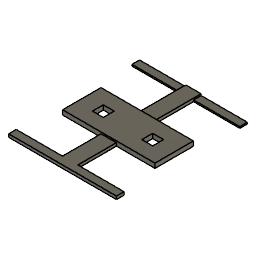
Ventilator Halterung andere Maße (Autodesk Fusion 360 design; units mm, degrees)
part number: 2026-08-07-16-50-58-000
Autodesk Fusion 360 part; units mm, degrees
sketch "Sketch1" plane through (0, 0, 0) normal (0, 0, 1) x (1, 0, 0)
  line L0 (0, 0) -> (60, 0)
  line L1 (60, 0) -> (60, 25)
  line L2 (60, 25) -> (0, 25)
  line L3 (0, 25) -> (0, 0)
  line L4 (5, 20) -> (55, 20)
  line L5 (55, 20) -> (55, 5)
  line L6 (55, 5) -> (5, 5)
  line L7 (5, 5) -> (5, 20)
  line L8 (10.5, 16) -> (17.5, 16)
  line L9 (17.5, 16) -> (17.5, 9)
  line L10 (17.5, 9) -> (10.5, 9)
  line L11 (10.5, 9) -> (10.5, 16)
  line L12 (42.5, 16) -> (49.5, 16)
  line L13 (49.5, 16) -> (49.5, 9)
  line L14 (49.5, 9) -> (42.5, 9)
  line L15 (42.5, 9) -> (42.5, 16)
  dimension "d1" = 60
  dimension "d2" = 25
  dimension "d3" = 50
  dimension "d4" = 15
  dimension "d5" = 5
  dimension "d7" = 5
  dimension "d8" = 7
  dimension "d9" = 7
  dimension "d10" = 4
  dimension "d12" = 7
  dimension "d13" = 7
  dimension "d15" = 4
  dimension "d16" = 5.5
  dimension "d17" = 5.5
  dimension "d18" = 25
  constraint horizontal L0
  constraint vertical L1
  constraint horizontal L2
  constraint vertical L3
  constraint coincident L0.start L3.end
  constraint horizontal L4
  constraint vertical L5
  constraint horizontal L6
  constraint vertical L7
  constraint horizontal L8
  constraint vertical L9
  constraint horizontal L10
  constraint vertical L11
  constraint horizontal L12
  constraint vertical L13
  constraint horizontal L14
  constraint vertical L15
  measures "d1" distance of L0.start L0.end
  measures "d2" distance of L0.start L2.end
  measures "d3" distance of L4.start L4.end
  measures "d4" distance of L4.start L6.end
  measures "d5" distance of L2 L4
  measures "d7" distance of L3 L7
  measures "d8" distance of L8.start L8.end
  measures "d9" distance of L8.start L10.end
  measures "d10" distance of L4 L8
  measures "d12" distance of L12.start L12.end
  measures "d13" distance of L12.start L14.end
  measures "d15" distance of L6 L14
  measures "d16" distance of L5 L13
  measures "d17" distance of L7 L11
  measures "d18" distance of L9 L15
sketch "Sketch2" plane through (0, 0, 0) normal (0, 0, 1) x (1, 0, 0)
extrude "Extrude1" add sketch "Sketch1" along normal blind 3 contours L0 L1 L2 L3 | L4 L5 L6 L7
sketch "Sketch3" plane through (0, 0, 0) normal (0, -1, 0) x (1, 0, 0)
  line L0 (0, 0) -> (60, 0)
  line L1 (60, 0) -> (60, 3)
  line L2 (60, 3) -> (0, 3)
  line L3 (0, 3) -> (0, 0)
  line L4 (25, 2) -> (35, 2)
  line L5 (35, 2) -> (35, 0)
  line L6 (35, 0) -> (25, 0)
  line L7 (25, 0) -> (25, 2)
  dimension "d21" = 10
  constraint horizontal L4
  constraint vertical L5
  constraint horizontal L6
  constraint vertical L7
  measures "d21" distance of L4.start L4.end
extrude "Extrude2" add sketch "Sketch3" along normal blind 30 contours L0 L4 L5 L6 L7
sketch "Sketch4" plane through (0, 25, 0) normal (0, 1, 0) x (-1, 0, 0)
  line L0 (-60, 0) -> (0, 0)
  line L1 (0, 0) -> (0, 3)
  line L2 (0, 3) -> (-60, 3)
  line L3 (-60, 3) -> (-60, 0)
  line L4 (-35, 2) -> (-25, 2)
  line L5 (-25, 2) -> (-25, 0)
  line L6 (-25, 0) -> (-35, 0)
  line L7 (-35, 0) -> (-35, 2)
  constraint horizontal L4
  constraint vertical L5
  constraint horizontal L6
  constraint vertical L7
  constraint coincident L0 L5.end
extrude "Extrude3" add sketch "Sketch4" along normal blind 30 contours L0 L4 L5 L6 L7
sketch "Sketch5" plane through (35, 0, 0) normal (1, 0, 0) x (0, 1, 0)
  line L0 (25, 2) -> (25, 0)
  line L1 (25, 0) -> (55, 0)
  line L2 (55, 0) -> (55, 2)
  line L3 (55, 2) -> (25, 2)
  line L4 (50, 1) -> (55, 1)
  line L5 (55, 1) -> (55, 0)
  line L6 (55, 0) -> (50, 0)
  line L7 (50, 0) -> (50, 1)
  constraint horizontal L4
  constraint vertical L5
  constraint horizontal L6
  constraint vertical L7
  constraint coincident L1.end L2.start
extrude "Extrude4" add sketch "Sketch5" along normal blind 30 contours L1 L2 L4 L5 L6 L7
sketch "Sketch6" plane through (25, 0, 0) normal (-1, 0, 0) x (0, -1, 0)
  line L0 (-25, 0) -> (-25, 2)
  line L1 (-25, 2) -> (-55, 2)
  line L2 (-55, 2) -> (-55, 0)
  line L3 (-55, 0) -> (-25, 0)
  line L4 (-50, 1) -> (-55, 1)
  line L5 (-55, 1) -> (-55, 0)
  line L6 (-55, 0) -> (-50, 0)
  line L7 (-50, 0) -> (-50, 1)
  constraint horizontal L4
  constraint vertical L5
  constraint horizontal L6
  constraint vertical L7
  constraint coincident L2.end L3.start
extrude "Extrude5" add sketch "Sketch6" along normal blind 30 contours L2 L3 L4 L5 L6 L7
sketch "Sketch7" plane through (35, 0, 0) normal (1, 0, 0) x (0, 1, 0)
  line L0 (0, 0) -> (0, 2)
  line L1 (0, 2) -> (-30, 2)
  line L2 (-30, 2) -> (-30, 0)
  line L3 (-30, 0) -> (0, 0)
  line L4 (-30, 2) -> (-25, 2)
  line L5 (-25, 2) -> (-25, 0)
  line L6 (-25, 0) -> (-30, 0)
  line L7 (-30, 0) -> (-30, 2)
  constraint horizontal L4
  constraint vertical L5
  constraint horizontal L6
  constraint vertical L7
  constraint coincident L3 L5.end
  constraint coincident L1.end L2.start
extrude "Extrude6" add sketch "Sketch7" along normal blind 30 contours L1 L2 L3 L4 L5 L6 L7
sketch "Sketch8" plane through (25, 0, 0) normal (-1, 0, 0) x (0, -1, 0)
  line L0 (0, 2) -> (0, 0)
  line L1 (0, 0) -> (30, 0)
  line L2 (30, 0) -> (30, 2)
  line L3 (30, 2) -> (0, 2)
  line L4 (25, 2) -> (30, 2)
  line L5 (30, 2) -> (30, 0)
  line L6 (30, 0) -> (25, 0)
  line L7 (25, 0) -> (25, 2)
  constraint horizontal L4
  constraint vertical L5
  constraint horizontal L6
  constraint vertical L7
  constraint coincident L1.end L2.start
  constraint coincident L3 L4.start
extrude "Extrude7" add sketch "Sketch8" along normal blind 30 contours L1 L2 L3 L4 L5 L6 L7
